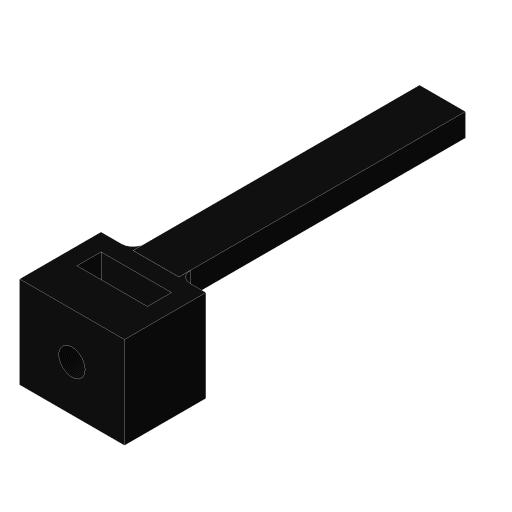
# Autodesk Inventor part: slider
Saved by Autodesk Inventor 2023 (Build 270158000, 158)
## iProperties
Created: 2024-01-18
Part Number: slider
Material: Generic
Document SubType Name: Modeling
Designer: qg3473
Density: 1 g/cm^3
Appearance: Gray
Author: qg3473
Autodesk Inventor part; units mm, degrees
ref_plane "YZ Plane" through (0, 0, 0) normal (1, 0, 0) x (0, 1, 0)
ref_plane "XZ Plane" through (0, 0, 0) normal (0, 1, 0) x (-1, 0, 0)
ref_plane "XY Plane" through (0, 0, 0) normal (0, 0, 1) x (1, 0, 0)
sketch "Sketch1" plane through (0, 0, 0) normal (0, 1, 0) x (-1, 0, 0)
  line L0 (-14.666, -11.6564) -> (-8.516, -11.6564)
  line L1 (-8.516, -11.6564) -> (-8.516, -13.7564)
  line L2 (-8.516, -13.7564) -> (-14.666, -13.7564)
  line L3 (-14.666, -13.7564) -> (-14.666, -11.6564)
  line L4 (-14.666, -11.6564) -> (-8.516, -13.7564) construction
  line L5 (-8.516, -11.6564) -> (-14.666, -13.7564) construction
  line L6 (-16.166, -15.2564) -> (-7.016, -15.2564)
  line L7 (-7.016, -15.2564) -> (-7.016, -10.1564)
  line L8 (-16.166, -10.1564) -> (-16.166, -15.2564)
  line L9 (-16.166, -8.1564) -> (-7.016, -8.1564)
  line L10 (-7.016, -10.1564) -> (-7.016, -8.1564)
  line L11 (-16.166, -10.1564) -> (-16.166, -8.1564)
  point P0 (0, 0)
  point P1 (-11.591, -12.7064)
  dimension "d0" = 6.15
  dimension "d1" = 2.1
  dimension "d2" = 1.5
  constraints: 24 end point, 3 parallel, 3 perpendicular, 2 midpoint, 1 horizontal, 1 other
  measures "d0" distance of L1.end L2.end
  measures "d1" distance of L0.end L1.end
  measures "d2" distance between parallel lines of L2 L6
extrude "Extrusion1" add sketch "Sketch1" along normal blind 8
sketch "Sketch4" plane through (7.016, 0, -8.1564) normal (0, 0, 1) x (1, 0, 0)
  circle A0 centre (4.5664, 4) radius 1.15
  point P0 (-7.016, 0)
  dimension "d13" = 2.3
  constraints: 1 centre point
  measures "d13" diameter of A0
extrude "Extrusion4" cut sketch "Sketch4" against normal blind 4
sketch "Sketch5" plane through (16.166, 0, -15.2564) normal (0, 0, -1) x (-1, 0, 0)
  line L0 (2.3524, 6.0027) -> (6.3524, 6.0027)
  line L1 (6.3524, 6.0027) -> (6.3524, 8.0027)
  line L2 (6.3524, 8.0027) -> (2.3524, 8.0027)
  line L3 (2.3524, 8.0027) -> (2.3524, 6.0027)
  line L4 (2.3524, 6.0027) -> (6.3524, 8.0027) construction
  line L5 (6.3524, 6.0027) -> (2.3524, 8.0027) construction
  point P0 (16.166, 0)
  point P1 (4.3524, 7.0027)
  dimension "d16" = 4
  dimension "d17" = 2
  constraints: 12 end point, 2 midpoint, 2 parallel, 1 horizontal, 1 perpendicular
  measures "d16" distance of L2.end L1.end
  measures "d17" distance of L1.end L0.end
extrude "Extrusion5" add sketch "Sketch5" along normal blind 25
fillet "Fillet1" radius 1 3 edges at (11.8136, 6.0027, -15.2564) (9.8136, 7.0014, -15.2564) (13.8136, 7.0014, -15.2564)
thread "Thread1" size "M0.6x0.15" class "6H" standard "ANSI Metric M Profile" full length
body "Solid1"
